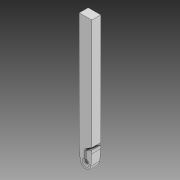
# Autodesk Inventor part: Winding_stick
Saved by Autodesk Inventor 2020 (Build 240168000, 168)
## iProperties
Created: 2021-03-13
Part Number: Winding_stick
Material: Generic
Document SubType Name: Modeling
Designer: DDeGo
Density: 1 g/cm^3
Appearance: Default
Author: DDeGo
Autodesk Inventor part; units mm, degrees
ref_plane "YZ Plane" through (0, 0, 0) normal (1, 0, 0) x (0, 1, 0)
ref_plane "XZ Plane" through (0, 0, 0) normal (0, 1, 0) x (-1, 0, 0)
ref_plane "XY Plane" through (0, 0, 0) normal (0, 0, 1) x (1, 0, 0)
sketch "Sketch1" plane through (0, 0, 0) normal (0, 0, 1) x (1, 0, 0)
  arc A0 (-0.4, 0.9165) -> (0.4, 0.9165) centre (0, 0) ccw
  arc A1 (-2.99, -0.2442) -> (2.99, -0.2442) centre (0, 0) ccw
  line L0 (-2.99, -0.2442) -> (-3.5, 6)
  line L1 (-3.5, 6) -> (-3.5, 71)
  line L2 (-3.5, 71) -> (3.5, 71)
  line L3 (3.5, 71) -> (3.5, 8.9445)
  line L4 (3.5, 6) -> (-3.5, 6) construction
  line L5 (3.5, 6) -> (2.99, -0.2442)
  line L6 (-0.4, 0.9165) -> (-0.4, 6.6928)
  line L7 (-0.4, 6.6928) -> (3.5, 8.9445)
  line L8 (3.5, 7.7898) -> (0.4, 6)
  line L9 (0.4, 6) -> (0.4, 0.9165)
  line L10 (0, 0) -> (0, 1.4678) construction
  line L11 (0, 1.4678) -> (-0.4, 1.4678) construction
  line L12 (0, 1.4678) -> (0.4, 1.4678) construction
  arc A2 (0, 1) -> (-0.4, 0.9165) centre (0, 0) ccw construction
  arc A3 (0.4, 0.9165) -> (0, 1) centre (0, 0) ccw construction
  line L13 (3.5, 8.9445) -> (3.5, 7.7898) construction
  line L14 (3.5, 7.7898) -> (3.5, 6)
  dimension "d0" = 2
  dimension "d1" = 0.8
  dimension "d2" = 1
  dimension "d3" = 30
  dimension "d4" = 2
  dimension "d5" = 7
  dimension "d6" = 6
  dimension "d7" = 65
  constraints: 30 end point, 8 point on circle, 6 perpendicular, 6 point on line, 4 centre point, 4 vertical, 2 coincident, 2 equal length, 2 tangent, 1 parallel
  measures "d0" diameter of A0
  measures "d1" distance between parallel lines of L9 L6
  measures "d2" distance between parallel lines of L8 L7
  measures "d3" angle of L4 L8
  measures "d4" radial gap between concentric circles of A1 A0
  measures "d5" distance of L4.start L0.end
  measures "d6" distance from line of point (0, 0) L4
  measures "d7" distance of L0.end L1.end
extrude "Extrusion1" add sketch "Sketch1" along normal blind 5
fillet "Fillet1" radius 1 3 edges at (0, -1, 5) (0, -1, 0) (0.4, 6, 2.5)
fillet "Fillet1" radius 2 1 edges at (-0.4, 6.6928, 2.5)
body "Solid1"
